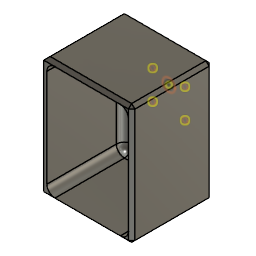
Onbox (Autodesk Fusion 360 design; units mm, degrees)
part number: 2026-08-24-00-09-28-916
Autodesk Fusion 360 part; units mm, degrees
sketch "Sketch1" plane through (0, 0, 0) normal (0, 1, 0) x (1, 0, 0)
  line L0 (-50.5, -50) -> (4, -50)
  line L1 (4, -50) -> (4, 24.5)
  line L2 (4, 24.5) -> (-50.5, 24.5)
  line L3 (-50.5, 24.5) -> (-50.5, -50)
  dimension "d1" = 74.5
  dimension "d2" = 54.5
  constraint perpendicular L0 L1
  constraint parallel L0 L2
  constraint parallel L1 L3
  constraint horizontal L0
  measures "d1" distance of L0.start L2.end
  measures "d2" distance of L1 L3
extrude "Extrude1" add sketch "Sketch1" along normal blind 50
shell "Shell1" thickness 2 removed faces 1 at (-14.1667, 0, 0.3333)
fillet "Fillet1" radius 5 1 edges at (-48.5, 24, -22.5)
fillet "Fillet2" radius 5 1 edges at (2, 24, -22.5)
fillet "Fillet3" radius 5 1 edges at (2, 24, 48)
fillet "Fillet4" radius 5 1 edges at (-48.5, 24, 48)
fillet "Fillet5" radius 5 8 edges at (-47.0355, 48, 46.5355) (-23.25, 48, 48) (0.5355, 48, 46.5355) (2, 48, 12.75) (0.5355, 48, -21.0355) (-23.25, 48, -22.5) (-47.0355, 48, -21.0355) (-48.5, 48, 12.75)
chamfer "Chamfer1" distance 2 angle 45 11 edges at (-50.5, 25, 50) (4, 25, 50) (4, 25, -24.5) (4, 50, 12.75) (4, 0, 12.75) (-23.25, 50, 50) (-23.25, 50, -24.5) (-50.5, 50, 12.75) (-50.5, 25, -24.5) (-23.25, 0, -24.5) (-23.25, 0, 50)
ref_plane "WorkPlane1" through (-23.25, 50, 12.75) normal (0, 1, 0) x (0, 0, 1)
sketch "Sketch2" plane through (0, 50, 0) normal (0, 1, 0) x (1, 0, 0)
  circle A0 centre (-22.9426, -23.5369) radius 4
  circle A1 centre (-22.9426, -23.5369) radius 3.5
  circle A2 centre (-32.9426, -9.5369) radius 1.5
  circle A3 centre (-12.9426, -9.5369) radius 1.5
  circle A4 centre (-12.9426, -27.5369) radius 1.5
  circle A5 centre (-32.9426, -27.5369) radius 1.5
extrude "Extrude2" add sketch "Sketch2" against normal blind 5 contours A2 | A3 | A4 | A5
extrude "Extrude3" cut sketch "Sketch2" against normal blind 7 contours A1
